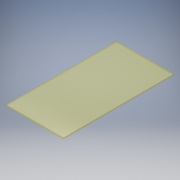
# Autodesk Inventor part: ControllerBoardTop
Saved by Autodesk Inventor 2019 (Build 230136000, 136)
## iProperties
Created: 2018-03-28
Part Number: ControllerBoardTop
Material: Polycarbonate, Clear
Document SubType Name: Modeling
Designer: james
Density: 1.2 g/cm^3
Appearance: Clear - Yellow
Mass: 203.712 g
Surface Area: 1100.4 cm^2
Volume: 169.76 cm^3
Author: james
Autodesk Inventor part; units mm, degrees
ref_plane "YZ Plane" through (0, 0, 0) normal (1, 0, 0) x (0, 1, 0)
ref_plane "XZ Plane" through (0, 0, 0) normal (0, 1, 0) x (-1, 0, 0)
ref_plane "XY Plane" through (0, 0, 0) normal (0, 0, 1) x (1, 0, 0)
sketch "Sketch1" plane through (0, 0, 0) normal (0, 1, 0) x (-1, 0, 0)
  line L0 (115.9067, 156.9125) -> (-61.8933, 156.9125)
  line L1 (-61.8933, 156.9125) -> (-61.8933, -185.9875)
  line L2 (-61.8933, -185.9875) -> (115.9067, -185.9875)
  line L3 (115.9067, -185.9875) -> (115.9067, 156.9125)
  point P0 (0, 0)
  dimension "d0" = 342.9
  dimension "d1" = 177.8
  constraints: 8 end point, 2 parallel, 1 horizontal, 1 perpendicular
  measures "d0" distance of L0.end L1.end
  measures "d1" distance of L0.start L0.end
extrude "Extrusion1" add sketch "Sketch1" along normal blind 3.175
body "Solid1"
